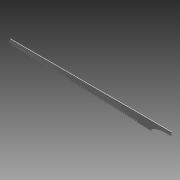
# Autodesk Inventor part: Saw blade
Saved by Autodesk Inventor 2015 (Build 190141000, 141)
## iProperties
Created: 2008-06-06
Part Number: Saw blade
Document SubType Name: Modeling
Designer: tangg
Density: 7.85 g/cm^3
Mass: 1.14139 g
Surface Area: 40.1035 cm^2
Volume: 1.14139 cm^3
Material: Alloy Steel
Appearance: Chrome - Polished
Author: tangg
Autodesk Inventor part; units mm, degrees
ref_plane "YZ Plane" through (0, 0, 0) normal (1, 0, 0) x (0, 1, 0)
ref_plane "XZ Plane" through (0, 0, 0) normal (0, 1, 0) x (-1, 0, 0)
ref_plane "XY Plane" through (0, 0, 0) normal (0, 0, 1) x (1, 0, 0)
sketch "Sketch1" plane through (0, 0, 0) normal (0, 0, 1) x (1, 0, 0)
  line L0 (0, 6.35) -> (-203.2, 6.35)
  line L1 (-203.2, 6.35) -> (-205.9496, 1.5875)
  line L2 (-203.2, 0) -> (-11.1125, -5.983)
  line L3 (-205.9496, 1.5875) -> (-203.2, 0)
  line L4 (0, 6.35) -> (16.7676, 6.35)
  line L5 (16.7676, 1.4388) -> (16.7676, 6.35)
  line L6 (16.7676, 1.4388) -> (7.9375, 1.3276)
  line L7 (-9.525, -3.175) -> (-11.1125, -5.983)
  arc A0 (7.9375, 1.3276) -> (-9.525, -3.175) centre (7.4648, -32.9526) ccw
  point P0 (0, 0)
  dimension "d2" = 120
  dimension "d3" = 203.2
  dimension "d6" = 6.35
  constraints: 16 end point, 2 point on circle, 1 centre point
  measures "d2" angle of L0 L1
  measures "d3" distance of L0.start L0.end
  measures "d6" distance from line of L0 L2.start
extrude "Extrusion3" add sketch "Sketch1" along normal mid plane 0.635
sketch "Sketch2" plane through (0, 0, 0) normal (0, 0, 1) x (1, 0, 0)
  line L0 (-31.869, -5.3365) -> (-31.8157, -2.7965)
  line L1 (-31.8157, -2.7965) -> (-29.3035, -5.4164)
  line L2 (-11.1125, -5.983) -> (-203.2, 0) projected
  point P0 (0, 0)
  dimension "d7" = 31.75
  dimension "d8" = 2.54
  dimension "d9" = 45
  constraints: 4 end point, 2 point on line
  measures "d7" distance from line of point (0, 0) L0
  measures "d8" vertical distance of L0.start L0.end
  measures "d9" angle of L1 L0
extrude "Extrusion4" cut sketch "Sketch2" against normal mid plane 3.175
pattern_linear "Rectangular Pattern1" count 55 spacing 3.175 along (-0.9995, 0.0311, 0) of "Extrusion4"
body "Solid1"
